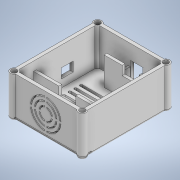
# Autodesk Inventor part: Part1
Saved by Autodesk Inventor 2021 (Build 250183000, 183)
## iProperties
Created: 2021-09-30
Part Number: Part1
Material: Generic
Document SubType Name: Modeling
Designer: david
Density: 1 g/cm^3
Appearance: Default
Author: david
## iProperties of the stored document _3DPrint.ipt
Created: 2021-09-30
Part Number: _3DPrint
Material: Generic
Document SubType Name: Modeling
Designer: david
Density: 1 g/cm^3
Appearance: Default
Author: david
Autodesk Inventor part; units mm, degrees
ref_plane "YZ Plane" through (0, 0, 0) normal (1, 0, 0) x (0, 1, 0)
ref_plane "XZ Plane" through (0, 0, 0) normal (0, 1, 0) x (-1, 0, 0)
ref_plane "XY Plane" through (0, 0, 0) normal (0, 0, 1) x (1, 0, 0)
sketch "Sketch1" plane through (0, 0, 0) normal (0, 1, 0) x (-1, 0, 0)
  line L0 (-29.25, -35.75) -> (29.25, -35.75)
  line L1 (29.25, -35.75) -> (29.25, 35.75)
  line L2 (29.25, 35.75) -> (-29.25, 35.75)
  line L3 (-29.25, 35.75) -> (-29.25, -35.75)
  line L4 (-29.25, -35.75) -> (29.25, 35.75) construction
  line L5 (29.25, -35.75) -> (-29.25, 35.75) construction
  point P0 (0, 0)
  dimension "d0" = 71.5
  dimension "d1" = 58.5
  constraints: 12 end point, 2 midpoint, 2 parallel, 1 horizontal, 1 perpendicular
  measures "d0" distance of L0.end L1.end
  measures "d1" distance of L1.end L2.end
extrude "Extrusion1" add sketch "Sketch1" along normal blind 33
shell "Shell1" thickness 3 outward yes removed faces 1 at (9.75, 33, 11.9167)
sketch "Sketch3" plane through (-29.25, 0, 35.75) normal (0, 1, 0) x (1, 0, 0)
  line L0 (58.5, 71.5) -> (58.5, 0) projected
  line L1 (0, 71.5) -> (0, 0) projected
  line L2 (58.5, 15) -> (0, 15)
  line L3 (0, 15) -> (0, 17.5)
  line L4 (0, 17.5) -> (58.5, 17.5)
  line L5 (58.5, 17.5) -> (58.5, 15)
  line L6 (58.5, 61.5) -> (18.5, 61.5)
  line L7 (18.5, 61.5) -> (18.5, 59)
  line L8 (18.5, 59) -> (58.5, 59)
  line L9 (58.5, 59) -> (58.5, 61.5)
  line L10 (58.5, 0) -> (0, 0) projected
  line L11 (58.5, 71.5) -> (0, 71.5) projected
  point P0 (29.25, 35.75)
  point P1 (0, 15)
  dimension "d5" = 2.5
  dimension "d6" = 40
  dimension "d7" = 2.5
  dimension "d61" = 15
  dimension "d62" = 41.5
  dimension "d63" = 10
  constraints: 16 end point, 4 parallel, 3 point on line, 2 horizontal, 2 perpendicular
  measures "d5" distance of L2.end L3.end
  measures "d6" distance of L8.end L7.end
  measures "d7" distance of L7.end L6.end
  measures "d61" distance between parallel lines of L10 L2
  measures "d62" distance between parallel lines of L8 L4
  measures "d63" distance between parallel lines of L11 L6
extrude "Extrusion2" add sketch "Sketch3" along normal blind 25 contours L0 L8 L7 L6 | L4 L0 L2 L1
sketch "Sketch5" plane through (-32.25, -3, 38.75) normal (0, 0, 1) x (1, 0, 0)
  circle A0 centre (31.8324, 18.68) radius 5
  circle A1 centre (31.8324, 18.68) radius 6
  circle A2 centre (31.8324, 18.68) radius 9
  circle A3 centre (31.8324, 18.68) radius 10
  circle A4 centre (31.8324, 18.68) radius 12.5
  circle A5 centre (31.8324, 18.68) radius 13.5
  line L0 (45.5583, 19.68) -> (18.1065, 19.68)
  line L1 (18.1065, 19.68) -> (18.1065, 17.68)
  line L2 (18.1065, 17.68) -> (45.5583, 17.68)
  line L3 (45.5583, 17.68) -> (45.5583, 19.68)
  line L4 (45.5583, 19.68) -> (18.1065, 17.68) construction
  line L5 (18.1065, 19.68) -> (45.5583, 17.68) construction
  line L6 (30.8324, 4.9541) -> (32.8324, 4.9541)
  line L7 (32.8324, 4.9541) -> (32.8324, 32.4059)
  line L8 (32.8324, 32.4059) -> (30.8324, 32.4059)
  line L9 (30.8324, 32.4059) -> (30.8324, 4.9541)
  line L10 (30.8324, 4.9541) -> (32.8324, 32.4059) construction
  line L11 (32.8324, 4.9541) -> (30.8324, 32.4059) construction
  line L12 (0, 0) -> (64.5, 0) projected
  point P0 (32.25, 3)
  point P1 (32.8324, 6.2201)
  point P2 (32.8324, 5.2171)
  point P3 (45.2953, 17.68)
  point P4 (44.2924, 17.68)
  point P5 (32.8324, 32.1429)
  point P6 (32.8324, 31.1399)
  point P7 (44.2924, 19.68)
  point P8 (45.2953, 19.68)
  point P9 (30.8324, 31.1399)
  point P10 (30.8324, 32.1429)
  point P11 (18.3695, 19.68)
  point P12 (19.3725, 19.68)
  point P13 (30.8324, 5.2171)
  point P14 (30.8324, 6.2201)
  point P15 (19.3725, 17.68)
  point P16 (18.3695, 17.68)
  point P17 (32.8324, 9.7357)
  point P18 (32.8324, 8.7301)
  point P19 (41.7823, 17.68)
  point P20 (40.7767, 17.68)
  point P21 (32.8324, 28.6299)
  point P22 (32.8324, 27.6243)
  point P23 (40.7767, 19.68)
  point P24 (41.7823, 19.68)
  point P25 (30.8324, 27.6243)
  point P26 (30.8324, 28.6299)
  point P27 (21.8825, 19.68)
  point P28 (22.8882, 19.68)
  point P29 (30.8324, 8.7301)
  point P30 (30.8324, 9.7357)
  point P31 (22.8882, 17.68)
  point P32 (21.8825, 17.68)
  point P33 (32.8324, 13.781)
  point P34 (32.8324, 12.7639)
  point P35 (37.7485, 17.68)
  point P36 (36.7314, 17.68)
  point P37 (32.8324, 24.5961)
  point P38 (32.8324, 23.579)
  point P39 (36.7314, 19.68)
  point P40 (37.7485, 19.68)
  point P41 (30.8324, 23.579)
  point P42 (30.8324, 24.5961)
  point P43 (25.9163, 19.68)
  point P44 (26.9334, 19.68)
  point P45 (30.8324, 12.7639)
  point P46 (30.8324, 13.781)
  point P47 (26.9334, 17.68)
  point P48 (25.9163, 17.68)
  dimension "d16" = 10
  dimension "d17" = 12
  dimension "d18" = 18
  dimension "d19" = 20
  dimension "d20" = 25
  dimension "d21" = 27
  dimension "d59" = 2
  dimension "d60" = 2
  dimension "d92" = 18.68
  constraints: 24 end point, 6 centre point, 5 coincident, 4 midpoint, 4 parallel, 2 horizontal, 2 perpendicular
  measures "d16" diameter of A0
  measures "d17" diameter of A1
  measures "d18" diameter of A2
  measures "d19" diameter of A3
  measures "d20" diameter of A4
  measures "d21" diameter of A5
  measures "d59" distance of L1.end L0.end
  measures "d60" distance of L8.end L7.end
  measures "d92" distance from line of L12 A0.centre
sketch "Sketch7" plane through (-29.25, 0, -35.75) normal (1, 0, 0) x (0, 0, -1)
  line L0 (-32, 15.5) -> (-21.5, 15.5)
  line L1 (-21.5, 15.5) -> (-21.5, 7)
  line L2 (-21.5, 7) -> (-32, 7)
  line L3 (-32, 7) -> (-32, 15.5)
  line L4 (0, 0) -> (-54, 0) projected
  point P0 (-35.75, 0)
  point P1 (-54, 25)
  point P2 (0, 33)
  dimension "d27" = 22
  dimension "d28" = 10.5
  dimension "d29" = 21.5
  dimension "d30" = 8.5
  dimension "d31" = 7
  constraints: 8 end point, 2 parallel, 1 horizontal, 1 perpendicular
  measures "d27" distance from line of point (-54, 25) L3
  measures "d28" distance between parallel lines of L1 L3
  measures "d29" distance from line of point (0, 33) L1
  measures "d30" distance between parallel lines of L0 L2
  measures "d31" distance from line of L2.end L4
extrude "Extrusion4" cut sketch "Sketch7" against normal up to surface (3 mm away)
extrude "Extrusion5" cut sketch "Sketch5" against normal up to surface (3 mm away) contours A0 L7 A1 L0 | L2 A1 L7 A0 | A0 L0 A1 L9 | A2 L7 A3 L0 | L9 A1 L2 A0 | L2 A3 L7 A2 | A2 L0 A3 L9 | A4 L7 A5 L0 | L9 A3 L2 A2 | L2 A5 L7 A4 | A4 L0 A5 L9 | L9 A5 L2 A4
sketch "Sketch9" plane through (0, -3, 0) normal (0, -1, 0) x (1, 0, 0)
  line L0 (-29.25, 35.75) -> (-29.25, -35.75) projected
  line L1 (24.9348, 11.6495) -> (-22.487, 11.6495)
  line L2 (-23.487, 10.6495) -> (-23.487, 10.4098)
  line L3 (-22.487, 9.4098) -> (24.9348, 9.4098)
  line L4 (25.9348, 10.4098) -> (25.9348, 10.6495)
  arc A0 (25.9348, 10.6495) -> (24.9348, 11.6495) centre (24.9348, 10.6495) ccw
  arc A1 (24.9348, 9.4098) -> (25.9348, 10.4098) centre (24.9348, 10.4098) ccw
  arc A2 (-22.487, 11.6495) -> (-23.487, 10.6495) centre (-22.487, 10.6495) ccw
  arc A3 (-23.487, 10.4098) -> (-22.487, 9.4098) centre (-22.487, 10.4098) ccw
  line L5 (24.9348, 6.6946) -> (-22.487, 6.6946)
  line L6 (-23.487, 5.6946) -> (-23.487, 5.4549)
  line L7 (-22.487, 4.4549) -> (24.9348, 4.4549)
  line L8 (25.9348, 5.4549) -> (25.9348, 5.6946)
  arc A4 (25.9348, 5.6946) -> (24.9348, 6.6946) centre (24.9348, 5.6946) ccw
  arc A5 (24.9348, 4.4549) -> (25.9348, 5.4549) centre (24.9348, 5.4549) ccw
  arc A6 (-22.487, 6.6946) -> (-23.487, 5.6946) centre (-22.487, 5.6946) ccw
  arc A7 (-23.487, 5.4549) -> (-22.487, 4.4549) centre (-22.487, 5.4549) ccw
  line L9 (24.9348, 1.8467) -> (-22.487, 1.8467)
  line L10 (-23.487, 0.8467) -> (-23.487, 0.6069)
  line L11 (-22.487, -0.3931) -> (24.9348, -0.3931)
  line L12 (25.9348, 0.6069) -> (25.9348, 0.8467)
  arc A8 (25.9348, 0.8467) -> (24.9348, 1.8467) centre (24.9348, 0.8467) ccw
  arc A9 (24.9348, -0.3931) -> (25.9348, 0.6069) centre (24.9348, 0.6069) ccw
  arc A10 (-22.487, 1.8467) -> (-23.487, 0.8467) centre (-22.487, 0.8467) ccw
  arc A11 (-23.487, 0.6069) -> (-22.487, -0.3931) centre (-22.487, 0.6069) ccw
  line L13 (24.9348, -3.4392) -> (-22.487, -3.4392)
  line L14 (-23.487, -4.4392) -> (-23.487, -4.6789)
  line L15 (-22.487, -5.6789) -> (24.9348, -5.6789)
  line L16 (25.9348, -4.6789) -> (25.9348, -4.4392)
  arc A12 (25.9348, -4.4392) -> (24.9348, -3.4392) centre (24.9348, -4.4392) ccw
  arc A13 (24.9348, -5.6789) -> (25.9348, -4.6789) centre (24.9348, -4.6789) ccw
  arc A14 (-22.487, -3.4392) -> (-23.487, -4.4392) centre (-22.487, -4.4392) ccw
  arc A15 (-23.487, -4.6789) -> (-22.487, -5.6789) centre (-22.487, -4.6789) ccw
  line L17 (24.9348, -8.4367) -> (-22.487, -8.4367)
  line L18 (-23.487, -9.4367) -> (-23.487, -9.6764)
  line L19 (-22.487, -10.6764) -> (24.9348, -10.6764)
  line L20 (25.9348, -9.6764) -> (25.9348, -9.4367)
  arc A16 (25.9348, -9.4367) -> (24.9348, -8.4367) centre (24.9348, -9.4367) ccw
  arc A17 (24.9348, -10.6764) -> (25.9348, -9.6764) centre (24.9348, -9.6764) ccw
  arc A18 (-22.487, -8.4367) -> (-23.487, -9.4367) centre (-22.487, -9.4367) ccw
  arc A19 (-23.487, -9.6764) -> (-22.487, -10.6764) centre (-22.487, -9.6764) ccw
  line L21 (24.9348, -13.4342) -> (-22.487, -13.4342)
  line L22 (-23.487, -14.4342) -> (-23.487, -14.6739)
  line L23 (-22.487, -15.6739) -> (24.9348, -15.6739)
  line L24 (25.9348, -14.6739) -> (25.9348, -14.4342)
  arc A20 (25.9348, -14.4342) -> (24.9348, -13.4342) centre (24.9348, -14.4342) ccw
  arc A21 (24.9348, -15.6739) -> (25.9348, -14.6739) centre (24.9348, -14.6739) ccw
  arc A22 (-22.487, -13.4342) -> (-23.487, -14.4342) centre (-22.487, -14.4342) ccw
  arc A23 (-23.487, -14.6739) -> (-22.487, -15.6739) centre (-22.487, -14.6739) ccw
  point P0 (-23.487, 9.4098)
  point P1 (-23.487, 4.4549)
  point P2 (-23.487, -0.3931)
  point P3 (-23.487, -5.6789)
  point P4 (-23.487, -10.6764)
  point P5 (-23.487, -15.6739)
  dimension "d93" = 1
  dimension "d94" = 1
  dimension "d95" = 1
  dimension "d96" = 1
  dimension "d97" = 1
  dimension "d98" = 1
  constraints: 48 end point, 48 point on circle, 48 tangent, 24 centre point, 18 equal radius, 12 parallel, 12 point on line, 6 horizontal, 6 perpendicular
  measures "d93" radius of A0
  measures "d94" radius of A4
  measures "d95" radius of A8
  measures "d96" radius of A12
  measures "d97" radius of A16
  measures "d98" radius of A20
extrude "Extrusion6" cut sketch "Sketch9" against normal blind 20
sketch "Sketch10" plane through (-29.25, 0, -35.75) normal (0, 1, 0) x (1, 0, 0)
  line L0 (18.5, -10) -> (58.5, -10) projected
  line L1 (0, 0) -> (58.5, 0) projected
  line L2 (40.5, -10) -> (52.5, -10)
  line L3 (52.5, -10) -> (52.5, 0)
  line L4 (52.5, 0) -> (40.5, 0)
  line L5 (40.5, 0) -> (40.5, -10)
  line L6 (58.5, 0) -> (58.5, -10) projected
  point P0 (29.25, -35.75)
  point P1 (40.5, 0)
  point P2 (52.5, -10)
  dimension "d43" = 6
  dimension "d44" = 12
  constraints: 8 end point, 2 parallel, 2 point on line, 1 horizontal, 1 perpendicular
  measures "d43" distance between parallel lines of L6 L3
  measures "d44" distance between parallel lines of L5 L3
extrude "Extrusion7" cut sketch "Sketch10" against normal up to surface (3 mm away) contours L5 L1 L3 L0
sketch "Sketch11" plane through (-29.25, 33, -35.75) normal (0, 0, 1) x (1, 0, 0)
  line L0 (40.5, -33) -> (0, -33) projected
  line L1 (29.5, -33) -> (40.5, -33)
  line L2 (40.5, -33) -> (40.5, -13)
  line L3 (40.5, -13) -> (29.5, -13)
  line L4 (29.5, -13) -> (29.5, -33)
  line L5 (58.5, -33) -> (58.5, 0) projected
  point P0 (29.25, -33)
  point P1 (58.5, -10)
  dimension "d47" = 20
  dimension "d48" = 18
  dimension "d49" = 11
  constraints: 8 end point, 2 parallel, 1 horizontal, 1 perpendicular, 1 point on line
  measures "d47" distance of L2.end L1.end
  measures "d48" distance from line of L5 L2.end
  measures "d49" distance between parallel lines of L2 L4
extrude "Extrusion8" cut sketch "Sketch11" against normal up to surface (3 mm away)
sketch "Sketch12" plane through (29.25, 0, 18.25) normal (0, 0, -1) x (-1, 0, 0)
  line L0 (0, 25) -> (58.5, 25) projected
  line L1 (21, 25) -> (36, 25)
  line L2 (36, 25) -> (36, 17)
  line L3 (36, 17) -> (21, 17)
  line L4 (21, 17) -> (21, 25)
  point P0 (29.25, 0)
  dimension "d52" = 8
  dimension "d53" = 15
  dimension "d57" = 21
  dimension "d58" = 22.5
  constraints: 8 end point, 2 parallel, 1 horizontal, 1 perpendicular
  measures "d52" distance between parallel lines of L3 L0
  measures "d53" distance between parallel lines of L2 L4
  measures "d57" distance from line of L0.start L4
  measures "d58" distance from line of L0.end L2
extrude "Extrusion9" cut sketch "Sketch12" against normal up to surface (2.5 mm away)
sketch "Sketch13" plane through (-10.75, 0, -23.25) normal (0, 0, 1) x (1, 0, 0)
  line L0 (0, 25) -> (40, 25) projected
  line L1 (16, 25) -> (31, 25)
  line L2 (31, 25) -> (31, 17)
  line L3 (31, 17) -> (16, 17)
  line L4 (16, 17) -> (16, 25)
  line L5 (0, 0) -> (0, 25) projected
  line L6 (40, 25) -> (40, 0) projected
  point P0 (10.75, 0)
  dimension "d64" = 15
  dimension "d65" = 8
  dimension "d66" = 16
  dimension "d67" = 9
  constraints: 8 end point, 2 parallel, 1 horizontal, 1 perpendicular, 1 point on line
  measures "d64" distance between parallel lines of L4 L2
  measures "d65" distance of L1.start L3.end
  measures "d66" distance between parallel lines of L4 L5
  measures "d67" distance between parallel lines of L6 L2
extrude "Extrusion10" cut sketch "Sketch13" against normal up to surface (2.5 mm away)
sketch "Sketch14" plane through (0, 33, 0) normal (0, 1, 0) x (1, 0, 0)
  circle A0 centre (-30.2315, -37.0138) radius 3.5
  circle A1 centre (30.232, -37.0138) radius 3.5
  circle A2 centre (-30.2315, 37.014) radius 3.5
  line L0 (-32.25, 38.75) -> (-32.25, -38.75) projected
  line L1 (-32.25, -38.75) -> (32.25, -38.75) projected
  line L2 (32.25, 38.75) -> (-32.25, 38.75) projected
  line L3 (32.25, -38.75) -> (32.25, 38.75) projected
  circle A3 centre (30.232, 37.014) radius 3.5
  point P0 (0, 0)
  dimension "d73" = 7
  dimension "d74" = 7
  dimension "d75" = 7
  dimension "d76" = 2.0185
  dimension "d77" = 1.7362
  dimension "d78" = 1.736
  dimension "d79" = 2.0185
  dimension "d80" = 2.018
  dimension "d81" = 1.7362
  dimension "d82" = 7
  dimension "d83" = 2.018
  dimension "d84" = 1.736
  constraints: 4 centre point
  measures "d73" diameter of A0
  measures "d74" diameter of A1
  measures "d75" diameter of A2
  measures "d76" distance from line of L0 A0.centre
  measures "d77" distance from line of L1 A0.centre
  measures "d78" distance from line of L2 A2.centre
  measures "d79" distance from line of L0 A2.centre
  measures "d80" distance from line of L3 A1.centre
  measures "d81" distance from line of L1 A1.centre
  measures "d82" diameter of A3
  measures "d83" distance from line of L3 A3.centre
  measures "d84" distance from line of L2 A3.centre
extrude "Extrusion11" add sketch "Sketch14" against normal up to surface (36 mm away) contours A0 L1 L0 | L0 L1 A0 | L0 L2 A2 | A2 L2 L0 | L1 L3 A1 | A1 L3 L1 | A3 L3 L2 | L2 L3 A3
sketch "Sketch15" plane through (0, 33, 0) normal (0, 1, 0) x (1, 0, 0)
  circle A0 centre (30.232, -37.0138) radius 2.45
  circle A1 centre (-30.2316, -37.0138) radius 2.45
  circle A2 centre (30.232, 37.014) radius 2.45
  circle A3 centre (-30.2315, 37.014) radius 2.445
  point P0 (0, 0)
  dimension "d85" = 4.9
  dimension "d86" = 4.9
  dimension "d87" = 4.9
  dimension "d88" = 4.89
  constraints: 4 centre point
  measures "d85" diameter of A0
  measures "d86" diameter of A1
  measures "d87" diameter of A2
  measures "d88" diameter of A3
extrude "Extrusion12" cut sketch "Sketch15" against normal blind 8
fillet "Fillet2" radius 2 8 edges at (32.25, -3, -0.0001) (0.0002, -3, 38.75) (32.586, -3, 39.604) (32.5859, -3, -39.6042) (0.0002, -3, -38.75) (-32.5852, -3, -39.6044) (-32.5853, -3, 39.6041) (-32.25, -3, -0.0001)
sketch "Sketch17" plane through (32.25, 33, 34.1541) normal (1, 0, 0) x (0, 0, -1)
  line L0 (0, 0) -> (0, -34) projected
  line L1 (-6.3597, 0) -> (-6.3597, -34) projected
  line L2 (0, -34) -> (-6.3597, -34)
  line L3 (-6.3597, -34) -> (-6.3597, -33.27)
  line L4 (-6.3597, -33.27) -> (0, -33.27)
  line L5 (0, -33.27) -> (0, -34)
  line L6 (-0.0003, -34) -> (68.3088, -34) projected
  line L7 (-0.0003, -34) -> (2.9997, -34)
  line L8 (2.9997, -34) -> (2.9997, -33.27)
  line L9 (2.9997, -33.27) -> (-0.0003, -33.27)
  line L10 (-0.0003, -33.27) -> (-0.0003, -34)
  point P0 (34.1541, -33)
  dimension "d101" = 0.73
  dimension "d102" = 3
  constraints: 16 end point, 4 parallel, 2 horizontal, 2 perpendicular, 1 point on line
  measures "d101" distance of L3.end L1.end
  measures "d102" distance of L9.end L8.end
extrude "Extrusion13" cut sketch "Sketch17" along normal blind 10 and the other way blind 60
sketch "Sketch18" plane through (27.1929, 33, -38.75) normal (0, 0, -1) x (-1, 0, 0)
  line L0 (37.9429, -33) -> (37.9429, -8) projected
  circle A0 centre (44.4113, -22.1048) radius 3.5
  point P0 (27.1929, -33)
  dimension "d107" = 7
  constraints: 1 centre point
  measures "d107" diameter of A0
extrude "Extrusion14" cut sketch "Sketch18" against normal up to surface (3 mm away)
sketch "Sketch19" plane through (11.25, -3, -35.75) normal (0, 0, 1) x (1, 0, 0)
  line L0 (-11.25, 3) -> (-13.25, 3)
  line L1 (-13.25, 3) -> (-13.25, 18)
  line L2 (-13.25, 18) -> (-11.25, 18)
  line L3 (-11.25, 18) -> (-11.25, 3)
  dimension "d110" = 2
  dimension "d111" = 15
  constraints: 8 end point, 2 parallel, 1 horizontal, 1 perpendicular
  measures "d110" distance of L1.end L2.end
  measures "d111" distance between parallel lines of L2 L0
extrude "Extrusion15" add sketch "Sketch19" along normal blind 5
sketch "Sketch20" plane through (-32.25, 33, -34.1547) normal (-1, 0, 0) x (0, 0, 1)
  line L0 (67.4707, -32.2867) -> (-28.9992, -32.2867) construction
  line L1 (-28.9992, -32.2867) -> (-28.9992, 55.9075) construction
  line L2 (-28.9992, 55.9075) -> (67.4707, 55.9075) construction
  line L3 (67.4707, 55.9075) -> (67.4707, -32.2867) construction
  line L4 (60.508, -32.0726) -> (57.209, -32.0726)
  line L5 (57.209, -32.0726) -> (57.209, -31.7157)
  spline S0 degree 2 poles (57.209, -31.7157) (58.6127, -31.5016) (58.6127, -27.0131) knots 0 0 0 1 1 1
  spline S1 degree 2 poles (58.6127, -27.0131) (58.6127, -25.4588) (58.7395, -24.1345) (59.5246, -22.9687) (61.1265, -22.2471) (62.2526, -22.2471) knots 0 0 0 1 2 3 4 4 4
  spline S2 degree 2 poles (62.2526, -22.2471) (63.4342, -22.2471) (65.0917, -22.937) (65.9719, -24.2376) (65.9719, -25.1892) knots 0 0 0 1 2 3 3 3
  line L6 (65.9719, -25.1892) -> (65.9719, -30.5262)
  spline S3 degree 2 poles (65.9719, -30.5262) (65.9719, -31.2558) (66.4874, -31.6999) (67.1139, -31.7157) knots 0 0 0 1 2 2 2
  line L7 (67.1139, -31.7157) -> (67.1139, -32.0726)
  line L8 (67.1139, -32.0726) -> (63.4422, -32.0726)
  line L9 (63.4422, -32.0726) -> (63.4422, -31.7157)
  spline S4 degree 2 poles (63.4422, -31.7157) (64.1083, -31.6999) (64.5841, -31.2161) (64.5841, -30.5262) knots 0 0 0 1 2 2 2
  line L10 (64.5841, -30.5262) -> (64.5841, -25.2526)
  spline S5 degree 2 poles (64.5841, -25.2526) (64.5841, -24.4993) (64.1162, -23.5159) (62.8633, -22.7229) (61.9275, -22.7229) knots 0 0 0 1 2 3 3 3
  spline S6 degree 2 poles (61.9275, -22.7229) (60.9997, -22.7229) (59.715, -23.397) (59.1361, -24.7451) (59.1361, -26.0932) knots 0 0 0 1 2 3 3 3
  spline S7 degree 2 poles (59.1361, -26.0932) (59.1361, -29.0591) (59.7546, -31.6444) (60.508, -31.7157) knots 0 0 0 1 2 2 2
  line L11 (60.508, -31.7157) -> (60.508, -32.0726)
  line L12 (56.6301, -32.0726) -> (54.0131, -32.0726)
  line L13 (54.0131, -32.0726) -> (54.0131, -31.7157)
  spline S8 degree 2 poles (54.0131, -31.7157) (54.2907, -31.7078) (54.2907, -31.462) knots 0 0 0 1 1 1
  spline S9 degree 2 poles (54.2907, -31.462) (54.2907, -31.3985) (54.259, -31.3113) knots 0 0 0 1 1 1
  line L14 (54.259, -31.3113) -> (51.872, -24.2613)
  line L15 (51.872, -24.2613) -> (50.619, -27.4176)
  spline S10 degree 2 poles (50.619, -27.4176) (50.0718, -28.8054) (50.0718, -30.0504) knots 0 0 0 1 1 1
  spline S11 degree 2 poles (50.0718, -30.0504) (50.0718, -31.6444) (51.3327, -31.7157) knots 0 0 0 1 1 1
  line L16 (51.3327, -31.7157) -> (51.3327, -32.0726)
  line L17 (51.3327, -32.0726) -> (48.6761, -32.0726)
  line L18 (48.6761, -32.0726) -> (48.6761, -31.7157)
  spline S12 degree 2 poles (48.6761, -31.7157) (48.9933, -31.7078) (48.9933, -31.4699) knots 0 0 0 1 1 1
  spline S13 degree 2 poles (48.9933, -31.4699) (48.9933, -31.4065) (48.9695, -31.3113) knots 0 0 0 1 1 1
  line L19 (48.9695, -31.3113) -> (46.5508, -24.2693)
  line L20 (46.5508, -24.2693) -> (45.0203, -28.1472)
  spline S14 degree 2 poles (45.0203, -28.1472) (44.3145, -29.9394) (44.3145, -30.7007) knots 0 0 0 1 1 1
  spline S15 degree 2 poles (44.3145, -30.7007) (44.3145, -31.2875) (44.8696, -31.6999) (45.5357, -31.7157) knots 0 0 0 1 2 2 2
  line L21 (45.5357, -31.7157) -> (45.5357, -32.0726)
  line L22 (45.5357, -32.0726) -> (42.1575, -32.0726)
  line L23 (42.1575, -32.0726) -> (42.1575, -31.7157)
  spline S16 degree 2 poles (42.1575, -31.7157) (42.5936, -31.7078) (43.3787, -30.669) (43.799, -29.6222) knots 0 0 0 1 2 2 2
  line L24 (43.799, -29.6222) -> (46.8046, -22.1043)
  line L25 (46.8046, -22.1043) -> (47.2566, -22.1043)
  line L26 (47.2566, -22.1043) -> (49.4295, -28.4564)
  spline S17 degree 2 poles (49.4295, -28.4564) (50.1591, -27.1559) (50.619, -25.9981) knots 0 0 0 1 1 1
  line L27 (50.619, -25.9981) -> (52.1495, -22.1043)
  line L28 (52.1495, -22.1043) -> (52.5857, -22.1043)
  line L29 (52.5857, -22.1043) -> (55.1154, -29.5746)
  spline S18 degree 2 poles (55.1154, -29.5746) (55.1789, -29.7411) (55.8371, -31.2558) (56.3605, -31.692) (56.6301, -31.7157) knots 0 0 0 1 2 3 3 3
  line L30 (56.6301, -31.7157) -> (56.6301, -32.0726)
  spline S19 degree 2 poles (40.508, -28.0837) (40.849, -28.4168) (41.2058, -29.1701) (41.2058, -29.5825) knots 0 0 0 1 2 2 2
  spline S20 degree 2 poles (41.2058, -29.5825) (41.2058, -30.661) (39.2154, -32.2867) (37.8752, -32.2867) knots 0 0 0 1 2 2 2
  spline S21 degree 2 poles (37.8752, -32.2867) (37.209, -32.2867) (36.0909, -31.9061) knots 0 0 0 1 1 1
  line L31 (36.0909, -31.9061) -> (36.0909, -29.5508)
  line L32 (36.0909, -29.5508) -> (36.638, -29.5508)
  spline S22 degree 2 poles (36.638, -29.5508) (36.7015, -30.5341) (37.7879, -31.7792) (38.573, -31.7792) knots 0 0 0 1 2 2 2
  spline S23 degree 2 poles (38.573, -31.7792) (39.2154, -31.7792) (40.056, -30.9941) (40.056, -30.3914) knots 0 0 0 1 2 2 2
  spline S24 degree 2 poles (40.056, -30.3914) (40.056, -29.8125) (39.6357, -29.3129) knots 0 0 0 1 1 1
  spline S25 degree 2 poles (39.6357, -29.3129) (39.2312, -28.8133) (37.669, -27.7586) knots 0 0 0 1 1 1
  spline S26 degree 2 poles (37.669, -27.7586) (36.4874, -26.9735) (36.0671, -26.4818) knots 0 0 0 1 1 1
  spline S27 degree 2 poles (36.0671, -26.4818) (35.6626, -25.9901) (35.6626, -25.2685) knots 0 0 0 1 1 1
  spline S28 degree 2 poles (35.6626, -25.2685) (35.6626, -24.0869) (37.8355, -22.2471) (39.2154, -22.2471) knots 0 0 0 1 2 2 2
  spline S29 degree 2 poles (39.2154, -22.2471) (40.1987, -22.2471) (41.4279, -22.715) knots 0 0 0 1 1 1
  line L33 (41.4279, -22.715) -> (41.4279, -25.4271)
  line L34 (41.4279, -25.4271) -> (40.8966, -25.4271)
  spline S30 degree 2 poles (40.8966, -25.4271) (40.8966, -24.2851) (39.5722, -22.7467) (38.6602, -22.7467) knots 0 0 0 1 2 2 2
  spline S31 degree 2 poles (38.6602, -22.7467) (37.8276, -22.7467) (36.8522, -23.7221) (36.8522, -24.4755) knots 0 0 0 1 2 2 2
  spline S32 degree 2 poles (36.8522, -24.4755) (36.8522, -25.1257) (37.2487, -25.6253) knots 0 0 0 1 1 1
  spline S33 degree 2 poles (37.2487, -25.6253) (37.6531, -26.1091) (39.0726, -27.0528) knots 0 0 0 1 1 1
  spline S34 degree 2 poles (39.0726, -27.0528) (39.8498, -27.5603) (40.508, -28.0837) knots 0 0 0 1 1 1
  point P0 (34.1547, -33)
  constraints: 2 other
emboss "Emboss3" sketch "Sketch20" operation cut depth 2 direction (1, 0, 0)
body "Solid1"
